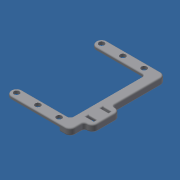
# Autodesk Inventor part: MotorServo2
Saved by Autodesk Inventor 2015 SP1 (Build 190203100, 203)
## iProperties
Created: 2015-11-11
Part Number: MotorServo2
Material: Generic
Document SubType Name: Modeling
Designer: Dale
Density: 1 g/cm^3
Appearance: Default
Author: Dale
Autodesk Inventor part; units mm, degrees
ref_plane "YZ Plane" through (0, 0, 0) normal (1, 0, 0) x (0, 1, 0)
ref_plane "XZ Plane" through (0, 0, 0) normal (0, 1, 0) x (-1, 0, 0)
ref_plane "XY Plane" through (0, 0, 0) normal (0, 0, 1) x (1, 0, 0)
sketch "Sketch1" plane through (0, 0, 0) normal (0, 0, 1) x (1, 0, 0)
  line L0 (-20.5, -32) -> (-20.5, -32)
  line L1 (-16.5, -28) -> (18, -28)
  line L2 (20, -26) -> (20, 26)
  line L3 (18, 28) -> (-16.5, 28)
  line L4 (-20.5, 32) -> (-20.5, 32)
  line L5 (-16.5, 36) -> (24, 36)
  line L6 (28, 32) -> (28, -2.3)
  line L7 (30, -4.3) -> (30, -4.3)
  line L8 (34, -8.3) -> (34, -21.3)
  line L9 (30, -25.3) -> (30, -25.3)
  line L10 (28, -27.3) -> (28, -32)
  line L11 (24, -36) -> (-16.5, -36)
  arc A0 (-20.5, -32) -> (-16.5, -36) centre (-16.5, -32) ccw
  arc A1 (24, -36) -> (28, -32) centre (24, -32) ccw
  arc A2 (-16.5, 36) -> (-20.5, 32) centre (-16.5, 32) ccw
  arc A3 (28, 32) -> (24, 36) centre (24, 32) ccw
  arc A4 (20, 26) -> (18, 28) centre (18, 26) ccw
  arc A5 (28, -2.3) -> (30, -4.3) centre (30, -2.3) ccw
  arc A6 (30, -25.3) -> (28, -27.3) centre (30, -27.3) ccw
  arc A7 (18, -28) -> (20, -26) centre (18, -26) ccw
  arc A8 (34, -8.3) -> (30, -4.3) centre (30, -8.3) ccw
  arc A9 (30, -25.3) -> (34, -21.3) centre (30, -21.3) ccw
  arc A10 (-16.5, -28) -> (-20.5, -32) centre (-16.5, -32) ccw
  arc A11 (-20.5, 32) -> (-16.5, 28) centre (-16.5, 32) ccw
  point P0 (0, 0)
  point P1 (-20.5, 28)
  point P2 (-20.5, 36)
  point P3 (28, -4.3)
  point P4 (34, -4.3)
  point P5 (28, -25.3)
  point P6 (28, -36)
  dimension "d0" = 72
  dimension "d1" = 36
  dimension "d2" = 48.5
  dimension "d3" = 40.5
  dimension "d5" = 20
  dimension "d6" = 8
  dimension "d7" = 8
  dimension "d8" = 6
  dimension "d9" = 10.7
  dimension "d11" = 4
  dimension "d12" = 2
  dimension "d13" = 4
  dimension "d14" = 4
  dimension "d53" = 21
  constraints: 24 end point, 24 point on circle, 24 tangent, 16 point on line, 12 centre point, 8 equal radius, 6 horizontal, 4 vertical
  measures "d0" distance between parallel lines of L11 L5
  measures "d1" distance from line of point (0, 0) L5
  measures "d2" distance between parallel lines of L6 L4
  measures "d3" distance between parallel lines of L2 L4
  measures "d5" distance from line of point (0, 0) L2
  measures "d6" distance between parallel lines of L11 L1
  measures "d7" distance between parallel lines of L3 L5
  measures "d8" distance of point (28, -4.3) point (34, -4.3)
  measures "d9" distance between parallel lines of L11 L9
  measures "d11" radius of A0
  measures "d12" radius of A4
  measures "d13" radius of A8
  measures "d14" radius of A10
  measures "d53" distance of L7.start L9.end
extrude "Base" add sketch "Sketch1" along normal blind 5.2
sketch "Sketch2" plane through (0, 0, 5.2) normal (0, 0, 1) x (1, 0, 0)
  circle A0 centre (-16.5, -32) radius 2.05
  line L0 (-16.5, -36) -> (24, -36) projected
  line L1 (34, -16) -> (34, -8.3) construction
  circle A1 centre (-0.5, -32) radius 2.05
  circle A2 centre (15.5, -32) radius 2.05
  circle A3 centre (-16.5, 32) radius 2.05
  circle A4 centre (-0.5, 32) radius 2.05
  circle A5 centre (15.5, 32) radius 2.05
  line L2 (-20.5, -28) -> (-20.5, -36) construction
  arc A6 (-16.5, -28) -> (-16.5, -36) centre (-16.5, -32) ccw projected
  point P0 (0, 0)
  dimension "d17" = 4.1
  dimension "d18" = 4
  dimension "d22" = 16
  dimension "d25" = 64
  dimension "d28" = 20
  dimension "d57" = 4
  constraints: 6 centre point, 4 end point, 3 vertical, 2 horizontal alignment, 1 horizontal, 1 tangent, 10 other
  measures "d17" diameter of A0
  measures "d18" distance from line of A0.centre L0
  measures "d22" distance of A0.centre A1.centre
  measures "d25" distance of A0.centre A3.centre
  measures "d28" distance from line of L1.start L0
  measures "d57" distance from line of L2 A0.centre
extrude "Mounting Holes" cut sketch "Sketch2" against normal through all
sketch "Sketch3" plane through (0, 0, 5.2) normal (0, 0, 1) x (1, 0, 0)
  line L0 (25, -19.3) -> (31, -19.3)
  line L1 (31, -19.3) -> (31, -21.3)
  line L2 (31, -21.3) -> (25, -21.3)
  line L3 (25, -21.3) -> (25, -19.3)
  line L4 (-16.5, -36) -> (24, -36) projected
  line L5 (20, 26) -> (20, -26) projected
  line L6 (25, -8.3) -> (31, -8.3)
  line L7 (31, -8.3) -> (31, -10.3)
  line L8 (31, -10.3) -> (25, -10.3)
  line L9 (25, -10.3) -> (25, -8.3)
  arc A0 (30, -25.3) -> (28, -27.3) centre (30, -27.3) ccw projected
  line L10 (24, 36) -> (-16.5, 36) projected
  point P0 (0, 0)
  dimension "d32" = 2
  dimension "d33" = 6
  dimension "d34" = 5
  dimension "d37" = 11
  dimension "d55" = 4
  constraints: 16 end point, 2 parallel, 1 horizontal, 1 perpendicular, 1 vertical, 8 other
  measures "d32" distance between parallel lines of L2 L0
  measures "d33" distance of L1.end L2.end
  measures "d34" distance between parallel lines of L3 L5
  measures "d37" distance of L0.start L6.start
  measures "d55" distance from line of L2 A0.start
extrude "Zip Tie Slot" cut sketch "Sketch3" against normal through all
sketch "Sketch4" plane through (0, 0, 0) normal (0, 0, -1) x (-1, 0, 0)
  line L0 (16.5, 36) -> (-24, 36) projected
  line L1 (-20, 36) -> (20.5, 36)
  line L2 (20.5, 36) -> (20.5, -36)
  line L3 (20.5, -36) -> (-20, -36)
  line L4 (-20, -36) -> (-20, 36)
  line L5 (-24, -36) -> (16.5, -36) projected
  line L6 (-20, -26) -> (-20, 26) projected
  arc A0 (16.5, 36) -> (16.5, 36) centre (16.5, 32) ccw projected
  point P0 (0, 0)
  point P1 (20, 40)
  constraints: 8 end point, 2 collinear, 2 parallel, 1 horizontal, 1 perpendicular, 1 point on line, 1 vertical, 1 other
extrude "Mount Cutout" cut sketch "Sketch4" against normal blind 3
sketch "Sketch5" plane through (0, 0, 0) normal (0, 0, -1) x (-1, 0, 0)
  line L0 (-31, -10.3) -> (-25, -10.3)
  line L1 (-25, -10.3) -> (-25, -19.3)
  line L2 (-25, -19.3) -> (-31, -19.3)
  line L3 (-31, -19.3) -> (-31, -10.3)
  line L4 (-25, -10.3) -> (-31, -10.3) projected
  line L5 (-31, -10.3) -> (-31, -8.3) projected
  point P0 (0, 0)
  constraints: 8 end point, 2 collinear, 2 parallel, 1 horizontal, 1 perpendicular
extrude "Zip Tie Cutout" cut sketch "Sketch5" against normal blind 2
fillet "Rounded Zip Tie Strap" radius 2 2 edges at (28, -19.3, 2) (28, -10.3, 2)
fillet "Rounded Cutout" radius 0.8 4 edges at (28, -8.3, 0) (31, -14.8, 0) (28, -21.3, 0) (25, -14.8, 0)
fillet "Rounded Top" radius 1 18 edges at (20, 0, 5.2) (19.4142, -27.4142, 5.2) (0.75, -28, 5.2) (-20.5, -32, 5.2) (3.75, -36, 5.2) (26.8284, -34.8284, 5.2) (28, -29.65, 5.2) (28.5858, -25.8858, 5.2) (32.8284, -24.1284, 5.2) (34, -14.8, 5.2) (32.8284, -5.4716, 5.2) (28.5858, -3.7142, 5.2) (28, 14.85, 5.2) (26.8284, 34.8284, 5.2) (3.75, 36, 5.2) (-20.5, 32, 5.2) (0.75, 28, 5.2) (19.4142, 27.4142, 5.2)
fillet "Rounded Bottom" radius 1 11 edges at (28, 14.85, 0) (26.8284, 34.8284, 0) (22, 36, 0) (28.5858, -3.7142, 0) (32.8284, -5.4716, 0) (34, -14.8, 0) (32.8284, -24.1284, 0) (28.5858, -25.8858, 0) (28, -29.65, 0) (26.8284, -34.8284, 0) (22, -36, 0)
fillet "Rounded Slots" radius 0.8 8 edges at (28, -8.3, 5.2) (31, -9.3, 5.2) (28, -10.3, 5.2) (25, -9.3, 5.2) (28, -19.3, 5.2) (28, -21.3, 5.2) (31, -20.3, 5.2) (25, -20.3, 5.2)
body "Solid1"
